Autodesk Fusion 360 part; units mm, degrees
(part 3 of 3)
sketch "Sketch1" plane through (0, 0, 0) normal (1, 0, 0) x (0, 0, -1)
  line L0 (12.9748, -104) -> (16.75, -107.7752)
  line L1 (18.5, -106.75) -> (17.8462, -106.75)
  line L2 (18.5, -93.25) -> (18.5, -97.5)
  line L3 (0, -102.5) -> (0, -110)
  line L4 (20, -110) -> (20, -102.5)
  line L5 (17.8462, -106.75) -> (14, -102.9038)
  line L6 (14, -102.9038) -> (14, -97.0962)
  line L7 (3.25, -108.5) -> (3.25, -107.7752)
  line L8 (0, -110) -> (7.5, -110)
  line L9 (7.5, -108.5) -> (3.25, -108.5)
  line L10 (7.0252, -104) -> (12.9748, -104)
  line L11 (16.75, -107.7752) -> (16.75, -108.5)
  line L12 (7.5, -110) -> (7.5, -108.5)
  line L13 (16.75, -108.5) -> (12.5, -108.5)
  line L14 (20, -102.5) -> (18.5, -102.5)
  line L15 (14, -97.0962) -> (17.8462, -93.25)
  line L16 (12.5, -110) -> (20, -110)
  line L17 (18.5, -102.5) -> (18.5, -106.75)
  line L18 (17.8462, -93.25) -> (18.5, -93.25)
  line L19 (7.0252, -96) -> (3.25, -92.2248)
  line L20 (20, -90) -> (12.5, -90)
  line L21 (0, -97.5) -> (1.5, -97.5)
  line L22 (2.1538, -93.25) -> (6, -97.0962)
  line L23 (1.5, -97.5) -> (1.5, -93.25)
  line L24 (16.75, -91.5) -> (16.75, -92.2248)
  line L25 (12.5, -90) -> (12.5, -91.5)
  line L26 (12.5, -91.5) -> (16.75, -91.5)
  line L27 (3.25, -92.2248) -> (3.25, -91.5)
  line L28 (3.25, -107.7752) -> (7.0252, -104)
  line L29 (12.9748, -96) -> (7.0252, -96)
  line L30 (1.5, -93.25) -> (2.1538, -93.25)
  line L31 (0, -90) -> (0, -97.5)
  line L32 (2.1538, -106.75) -> (1.5, -106.75)
  line L33 (1.5, -106.75) -> (1.5, -102.5)
  line L34 (12.5, -108.5) -> (12.5, -110)
  line L35 (6, -97.0962) -> (6, -102.9038)
  line L36 (7.5, -90) -> (0, -90)
  line L37 (7.5, -91.5) -> (7.5, -90)
  line L38 (3.25, -91.5) -> (7.5, -91.5)
  line L39 (16.75, -92.2248) -> (12.9748, -96)
  line L40 (18.5, -97.5) -> (20, -97.5)
  line L41 (20, -97.5) -> (20, -90)
  line L42 (1.5, -102.5) -> (0, -102.5)
  line L43 (6, -102.9038) -> (2.1538, -106.75)
  circle A0 centre (10, -100) radius 2.15
  line L44 (16.75, -91.5) -> (3.25, -91.5) construction
  line L45 (3.25, -91.5) -> (3.25, -92.2248)
  line L46 (3.25, -92.2248) -> (7.0252, -96)
  line L47 (12.9748, -96) -> (7.0252, -96)
  line L48 (12.9748, -96) -> (16.75, -92.2248)
  line L49 (16.75, -92.2248) -> (16.75, -91.5)
  line L50 (12.5, -91.5) -> (12.5, -90)
  line L51 (7.5, -91.5) -> (7.5, -90)
  line L52 (12.5, -90) -> (20, -90)
  line L53 (20, -90) -> (20, -88)
  line L54 (20, -88) -> (0, -88)
  line L55 (0, -88) -> (0, -90)
  line L56 (0, -90) -> (7.5, -90)
  line L57 (7.5, -90) -> (7.7, -90)
  line L58 (7.7, -90) -> (7.7, -91.5)
  line L59 (3.25, -92.2248) -> (3.3914, -92.0834) construction
  line L60 (3.25, -91.5) -> (3.3914, -91.6414) construction
  line L61 (3.25, -91.5) -> (3.45, -91.5) construction
  line L62 (3.3914, -91.6414) -> (3.3914, -92.0834)
  line L63 (3.3914, -91.6414) -> (7.7, -91.6414)
  line L64 (7.7, -91.6414) -> (7.7, -91.5)
  line L65 (7.0252, -96) -> (7.1666, -95.8586) construction
  line L66 (3.3914, -92.0834) -> (7.1666, -95.8586)
  line L67 (7.1666, -95.8586) -> (10, -95.8586)
  line L68 (10, -95.8586) -> (10, -91.5) construction
  line L69 (16.6086, -91.6414) -> (12.3, -91.6414)
  line L70 (16.6086, -91.6414) -> (16.6086, -92.0834)
  line L71 (16.6086, -92.0834) -> (12.8334, -95.8586)
  line L72 (12.3, -90) -> (12.3, -91.5)
  line L73 (12.5, -90) -> (12.3, -90)
  line L74 (12.8334, -95.8586) -> (10, -95.8586)
  line L75 (12.3, -91.6414) -> (12.3, -91.5)
  dimension "d1" = 0.2
  dimension "d4" = 0.2
  dimension "d5" = 45
  dimension "d6" = 0.2
  dimension "d7" = 0.2
  constraint perpendicular L37 L57
  constraint coincident L44 L58.end
  constraint perpendicular L44 L58
  constraint perpendicular L46 L59
  constraint horizontal L61
  constraint perpendicular L58 L63
  constraint perpendicular L44 L64
  constraint perpendicular L19 L65
  constraint parallel L47 L67
  constraint midpoint L44 L68.end
  constraint perpendicular L44 L68
  constraint symmetric L36.start L68 L20.end
  constraint symmetric L57.end L68 L72.start
  constraint symmetric L58.end L68 L72.end
  constraint symmetric L59.end L68 L70.end
  constraint symmetric L60.end L68 L69.start
  constraint symmetric L63.end L68 L69.end
  constraint symmetric L65.end L68 L71.end
  constraint symmetric L67.end L68 L74.end
  measures "d1" distance of L36.start L57.end
  measures "d4" distance of L19.end L59.end
  measures "d5" angle of L60 L61
  measures "d6" distance of L27.end L60.end
  measures "d7" distance of L19.start L65.end
extrude "Extrude1" add sketch "Sketch1" along normal blind 300 contours L20 L36 L52 L53 L54 L55 L56 L57 L58 L62 L63 L64 L66 L67 L69 L70 L71 L72 L73 L74 L75
extrude "Extrude2" add 1 faces at (100, -88, -13.3333) along direction (0, 1, 0) blind 1.482
extrude "Extrude3" cut 1 faces at (100, -86.518, -13.3333) along direction (0, -1, 0) blind 0.82
sketch "Sketch2" plane through (0, -87.338, 0) normal (0, 1, 0) x (-1, 0, 0)
  line L0 (0, -20) -> (0, 0)
  line L1 (0, 0) -> (-300, 0)
  line L2 (-300, 0) -> (-300, -20)
  line L3 (-300, -20) -> (0, -20)
  line L4 (0, 0) -> (0, -5)
  line L5 (0, -5) -> (-300, -5)
  line L6 (0, -5) -> (0, -15)
  line L7 (0, -15) -> (-300, -15)
  line L8 (-300, -15) -> (-300, -5)
  dimension "d14" = 5
  dimension "d15" = 300
  dimension "d16" = 10
  dimension "d17" = 300
  constraint coincident L0.end L1.start
  constraint perpendicular L3 L4
  constraint perpendicular L4 L5
  constraint perpendicular L5 L6
  constraint perpendicular L6 L7
  measures "d14" distance of L0.end L4.end
  measures "d15" distance of L4.end L5.end
  measures "d16" distance of L4.end L6.end
  measures "d17" distance of L6.end L7.end
extrude "Extrude4" cut sketch "Sketch2" against normal blind 2.662 contours L0 L2 L3 L7 | L0 L1 L2 L4 L5
